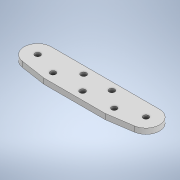
# Autodesk Inventor part: prig to kauri conversion plate
Saved by Autodesk Inventor 2020 (Build 240168000, 168)
## iProperties
Created: 2022-05-24
Part Number: prig to kauri conversion plate
Material: Generic
Document SubType Name: Modeling
Designer: Steven
Density: 1 g/cm^3
Appearance: Default
Author: Steven
Autodesk Inventor part; units mm, degrees
ref_plane "YZ Plane" through (0, 0, 0) normal (1, 0, 0) x (0, 1, 0)
ref_plane "XZ Plane" through (0, 0, 0) normal (0, 1, 0) x (-1, 0, 0)
ref_plane "XY Plane" through (0, 0, 0) normal (0, 0, 1) x (1, 0, 0)
sketch "Sketch1" plane through (0, 0, 0) normal (0, 1, 0) x (-1, 0, 0)
  arc A0 (-35.8309, 5.9248) -> (-30.0072, 12.1625) centre (-41.895, 17.4238) ccw construction
  arc A1 (-35.8309, 5.9248) -> (-21.1612, -13.9708) centre (-30, -5.1319) ccw construction
  line L0 (-21.1612, -13.9708) -> (-13.9152, -6.7248) construction
  arc A2 (-13.9152, -6.7248) -> (-11.0366, -3.464) centre (-38.6639, 18.024) ccw construction
  line L1 (-11.0366, -3.464) -> (-3.1574, 6.6664) construction
  arc A3 (3.1574, 6.6664) -> (-3.1574, 6.6664) centre (0, 4.2106) ccw construction
  line L2 (3.1574, 6.6664) -> (11.0366, -3.464) construction
  arc A4 (11.0366, -3.464) -> (13.9152, -6.7248) centre (38.6639, 18.024) ccw construction
  line L3 (13.9152, -6.7248) -> (21.1612, -13.9708) construction
  arc A5 (21.1612, -13.9708) -> (35.8309, 5.9248) centre (30, -5.1319) ccw construction
  arc A6 (30.0072, 12.1625) -> (35.8309, 5.9248) centre (41.895, 17.4238) ccw construction
  circle A7 centre (25.4558, 7.8975) radius 1.5 construction
  circle A8 centre (-16.9706, -0.5878) radius 1.5
  circle A9 centre (16.9706, -0.5878) radius 1.5
  circle A10 centre (-25.4558, 7.8975) radius 1.5 construction
  circle A11 centre (30, -5.1319) radius 1.5
  circle A12 centre (-30, -5.1319) radius 1.5
  circle A13 centre (16.9706, -0.5878) radius 5 construction
  circle A14 centre (-16.9706, -0.5878) radius 5 construction
  arc A15 (-31.1155, 2.2846) -> (-30, -12.6319) centre (-30, -5.1319) ccw
  arc A16 (30, -12.6319) -> (31.1155, 2.2846) centre (30, -5.1319) ccw
  line L4 (30, -12.6319) -> (-30, -12.6319)
  line L5 (-16.9706, 4.4122) -> (16.9706, 4.4122)
  line L6 (-16.9706, 4.4122) -> (-31.1155, 2.2846)
  line L7 (16.9706, 4.4122) -> (31.1155, 2.2846)
  arc A17 (31.1155, 2.2846) -> (30, -12.6319) centre (30, -5.1319) ccw construction
  arc A18 (-30, -12.6319) -> (-31.1155, 2.2846) centre (-30, -5.1319) ccw construction
  line L8 (0, 4.2106) -> (0, -4.2106) construction
  line L9 (0, -4.2106) -> (3.1574, -4.2106) construction
  line L10 (0, -4.2106) -> (0, -12.6319) construction
  circle A19 centre (0, 0) radius 1.55
  line L11 (0, -8.4213) -> (15.6117, -8.4213) construction
  line L12 (13.9152, -6.7248) -> (21.1612, -13.9708)
  line L13 (0, -8.4213) -> (-15.6117, -8.4213) construction
  line L14 (-21.1612, -13.9708) -> (-13.9152, -6.7248)
  circle A20 centre (7.8058, -8.4213) radius 1.55
  circle A21 centre (-7.8058, -8.4213) radius 1.55
  point P0 (0, 0)
  point P1 (-15, 9.8681)
  point P2 (15, 9.8681)
  dimension "d0" = 10
  dimension "d1" = 10
  dimension "d2" = 15
  dimension "d3" = 15
  dimension "d4" = 3.1
  dimension "d5" = 3.1
  dimension "d6" = 3.1
  constraints: 30 end point, 22 point on circle, 20 centre point, 5 midpoint, 4 coincident, 4 horizontal, 3 point on line, 3 tangent, 2 vertical alignment, 4 other
  measures "d2" diameter of A15
  measures "d3" diameter of A16
  measures "d4" diameter of A19
  measures "d5" diameter of A20
  measures "d6" diameter of A21
extrude "Extrusion1" add sketch "Sketch1" along normal blind 3
body "Solid1"
